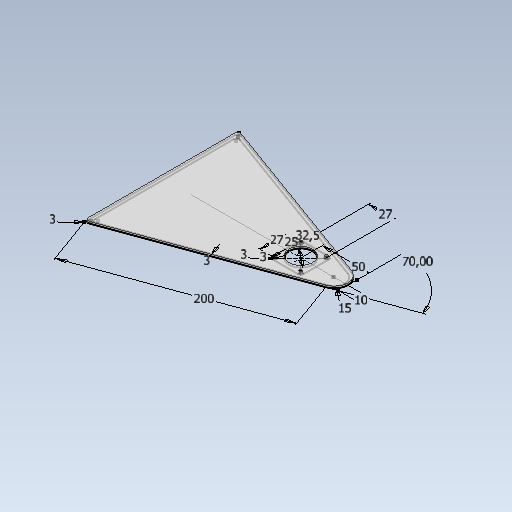
# Autodesk Inventor part: PRTGN_baseipt
Saved by Autodesk Inventor 2026.2 (Build 302298000, 298)
## iProperties
Created: 2026-05-31
Part Number: PRTGN_baseipt
Material: Generic
Document SubType Name: Modeling
Designer: MenMe
Density: 1 g/cm^3
Appearance: Default
Author: MenMe
Autodesk Inventor part; units mm, degrees
ref_plane "YZ Plane" through (0, 0, 0) normal (1, 0, 0) x (0, 1, 0)
ref_plane "XZ Plane" through (0, 0, 0) normal (0, 1, 0) x (-1, 0, 0)
ref_plane "XY Plane" through (0, 0, 0) normal (0, 0, 1) x (1, 0, 0)
sketch "Sketch1" plane through (0, 0, 0) normal (0, 1, 0) x (-1, 0, 0)
  line L0 (0, 0) -> (0, -0.5031)
  line L1 (9.8697, 13.5923) -> (193.7822, 80.5309)
  line L2 (166.1465, 0) -> (0, 0) construction
  line L3 (0, 0) -> (0, 0.5031)
  line L4 (9.8697, -13.5923) -> (193.7822, -80.5309)
  circle A0 centre (50, 0) radius 12.5
  circle A1 centre (63.5, 13.5) radius 1.5
  circle A2 centre (63.5, -13.5) radius 1.5
  circle A3 centre (36.5, 13.5) radius 1.5
  circle A4 centre (36.5, -13.5) radius 1.5
  line L5 (63.5, 13.5) -> (36.5, -13.5) construction
  line L6 (36.5, 13.5) -> (63.5, -13.5) construction
  arc A5 (9.8697, 13.5923) -> (0, -0.5031) centre (15, -0.5031) ccw
  arc A6 (0, 0.5031) -> (9.8697, -13.5923) centre (15, 0.5031) ccw
  line L7 (63.25, 16.25) -> (36.75, 16.25)
  line L8 (33.75, 13.25) -> (33.75, -13.25)
  line L9 (36.75, -16.25) -> (63.25, -16.25)
  line L10 (66.25, -13.25) -> (66.25, 13.25)
  line L11 (66.25, 16.25) -> (33.75, -16.25) construction
  line L12 (33.75, 16.25) -> (66.25, -16.25) construction
  arc A7 (66.25, 13.25) -> (63.25, 16.25) centre (63.25, 13.25) ccw
  arc A8 (63.25, -16.25) -> (66.25, -13.25) centre (63.25, -13.25) ccw
  arc A9 (33.75, -13.25) -> (36.75, -16.25) centre (36.75, -13.25) ccw
  arc A10 (36.75, 16.25) -> (33.75, 13.25) centre (36.75, 13.25) ccw
  line L13 (197.8082, 77.7119) -> (197.8082, -77.7119)
  line L14 (190.7822, 76.2465) -> (10.8958, 10.7732)
  arc A11 (10.8958, 10.7732) -> (3, -0.5031) centre (15, -0.5031) ccw
  line L15 (3, -0.5031) -> (3, 0)
  line L16 (3, 0) -> (3, 0.5031)
  arc A12 (3, 0.5031) -> (10.8958, -10.7732) centre (15, 0.5031) ccw
  line L17 (10.8958, -10.7732) -> (190.7822, -76.2465)
  line L18 (194.8082, -73.4274) -> (194.8082, 73.4274)
  arc A13 (197.8082, 77.7119) -> (193.7822, 80.5309) centre (194.8082, 77.7119) ccw
  arc A14 (194.8082, 73.4274) -> (190.7822, 76.2465) centre (191.8082, 73.4274) ccw
  arc A15 (190.7822, -76.2465) -> (194.8082, -73.4274) centre (191.8082, -73.4274) ccw
  arc A16 (193.7822, -80.5309) -> (197.8082, -77.7119) centre (194.8082, -77.7119) ccw
  point P0 (0, 10)
  point P1 (197.8082, 81.9963)
  point P2 (0, -10)
  point P3 (197.8082, -81.9963)
  point P4 (50, 0)
  point P5 (194.8082, 77.7119)
  point P6 (194.8082, -77.7119)
  point P7 (0.0084, 0)
  point P8 (3.0106, 0)
  dimension "d1" = 25
  dimension "d2" = 50
  dimension "d3" = 27
  dimension "d4" = 27
  dimension "d5" = 3
  dimension "d6" = 15
  dimension "d7" = 10
  dimension "d9" = 70
  dimension "d10" = 32.5
  dimension "d11" = 3
  dimension "d12" = 200
  dimension "d13" = 3
  dimension "d20" = 3
  constraints: 38 end point, 24 point on circle, 21 point on line, 20 tangent, 17 centre point, 10 equal radius, 3 midpoint, 2 horizontal, 2 horizontal alignment, 2 parallel, 2 symmetric about line, 2 vertical, 2 vertical alignment, 1 collinear, 1 perpendicular, 6 other
  measures "d1" diameter of A0
  measures "d2" distance from line of L3 A0.centre
  measures "d3" distance of L6.end L5.start
  measures "d4" distance of L5.end L6.end
  measures "d5" diameter of A1
  measures "d6" radius of A5
  measures "d7" distance of point (0, 10) L0.start
  measures "d9" angle of L0 L1
  measures "d10" distance between parallel lines of L9 L7
  measures "d11" radius of A7
  measures "d12" distance of point (197.808, 81.996) L1.start
  measures "d13" distance between parallel lines of L1 L14
  measures "d20" radius of A13
extrude "Extrusion1" add sketch "Sketch1" along normal blind 2 contours A5 L1 A13 L13 A16 L4 A6 | A0 | A1 | A2 | A3 | A4 | A7 L10 A8 L9 A9 L8 A10 L7 | A14 L18 A15 L17 A12 A11 L14 | A11 L15 L16 A12
extrude "Extrusion2" cut sketch "Sketch1" along normal blind 2 contours A0 | A1 | A2 | A3 | A4
body "Solid1"
